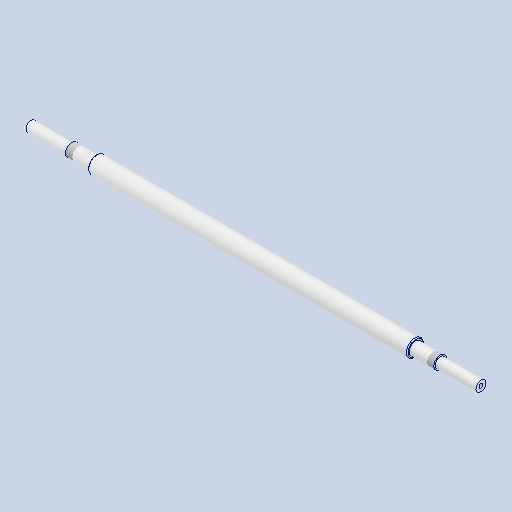
# Autodesk Inventor part: P301
Saved by Autodesk Inventor 2023 (Build 270158000, 158)
## iProperties
Created: 2022-08-24
Part Number: P301
Material: Aluminum 6061
Document SubType Name: Modeling
Designer: D.C. Eksteen
Density: 2.7 g/cm^3
Appearance: Aluminum - Flat
Description: FRONT ROLLER SHAFT
Author: D.C. Eksteen
Title: IDLE ROLLER SHAFT
Autodesk Inventor part; units mm, degrees
ref_plane "YZ Plane" through (0, 0, 0) normal (1, 0, 0) x (0, 1, 0)
ref_plane "XZ Plane" through (0, 0, 0) normal (0, 1, 0) x (-1, 0, 0)
ref_plane "XY Plane" through (0, 0, 0) normal (0, 0, 1) x (1, 0, 0)
sketch "Sketch1" plane through (0, 0, 0) normal (0, 0, 1) x (1, 0, 0)
  line L0 (0, 0) -> (0, 10)
  line L1 (0, 10) -> (188, 10)
  line L2 (188, 10) -> (188, 7.5)
  line L3 (188, 7.5) -> (195, 7.5)
  line L4 (195, 7.5) -> (195, 7.5)
  line L5 (195, 7.5) -> (217, 7.5)
  line L6 (265, 0) -> (0, 0)
  line L7 (217, 7.5) -> (217, 6)
  line L8 (217, 6) -> (265, 6)
  line L9 (265, 6) -> (265, 0)
  line L10 (0, 10) -> (-188, 10)
  line L11 (-188, 10) -> (-188, 7.5)
  line L12 (-188, 7.5) -> (-195, 7.5)
  line L13 (-195, 7.5) -> (-195, 7.5)
  line L14 (-195, 7.5) -> (-217, 7.5)
  line L15 (-265, 0) -> (0, 0)
  line L16 (-217, 7.5) -> (-217, 6)
  line L17 (-217, 6) -> (-265, 6)
  line L18 (-265, 6) -> (-265, 0)
  point P0 (188, 8.75)
  point P1 (217, 6.75)
  point P2 (-188, 8.75)
  point P3 (-217, 6.75)
  dimension "d0" = 10
  dimension "d1" = 188
  dimension "d2" = 7
  dimension "d4" = 265
  dimension "d5" = 6
  dimension "d6" = 7.5
  dimension "d7" = 7.5
  dimension "d12" = 217
  constraints: 38 end point, 10 symmetric about line, 7 perpendicular, 2 midpoint, 2 vertical, 1 horizontal
  measures "d0" distance of L0.start L0.end
  measures "d1" distance of L0.end L1.end
  measures "d2" distance of L2.end L3.end
  measures "d4" distance between parallel lines of L0 L9
  measures "d5" distance between parallel lines of L6 L8
  measures "d6" distance between parallel lines of L6 L5
  measures "d7" distance between parallel lines of L6 L3
  measures "d12" distance between parallel lines of L0 L7
revolve "Revolution1" add sketch "Sketch1" angle 360 about axis through (265, 0, 0) along (-1, 0, 0)
chamfer "Chamfer1" distance 1 angle 45 2 edges at (188, -10, 0) (-188, -10, 0)
thread "Thread1" size "M15x1.5" class "6g" standard "ANSI Metric M Profile" length 8
thread "Thread2" size "M15x1.5" class "6g" standard "ANSI Metric M Profile" length 8
sketch "Sketch3" plane through (-265, 0, 0) normal (-1, 0, 0) x (0, 0, 1)
  point P0 (0, 0)
  point P1 (0, 0)
  constraints: 1 coincident
hole "Hole1" at (-265, 0, 0) direction (1, 0, 0) diameter 4.917 depth 17.1 tip angle 118 thread size "M6x1" class "6H" standard "ISO Metric profile"
sketch "Sketch4" plane through (265, 0, 0) normal (1, 0, 0) x (0, 0, -1)
  point P0 (0, 0)
  point P1 (0, 0)
  constraints: 1 coincident
hole "Hole2" at (265, 0, 0) direction (-1, 0, 0) diameter 4.917 depth 17.1 tip angle 118 thread size "M6x1" class "6H" standard "ISO Metric profile"
body "Solid1"
